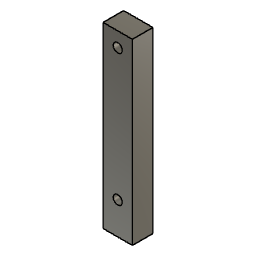
link2 v3 (Autodesk Fusion 360 design; units mm, degrees)
Autodesk Fusion 360 part; units mm, degrees
sketch "Sketch1" plane through (0, 0, 0) normal (0, 1, 0) x (1, 0, 0)
  line L0 (5, 27.5) -> (-5, 27.5)
  line L1 (-5, 27.5) -> (-5, -27.5)
  line L2 (-5, -27.5) -> (5, -27.5)
  line L3 (5, -27.5) -> (5, 27.5)
  line L4 (5, 27.5) -> (-5, -27.5) construction
  line L5 (-5, 27.5) -> (5, -27.5) construction
  line L6 (0, -24.05) -> (0, -22.5)
  circle A0 centre (0, -22.5) radius 1.55
  circle A1 centre (0, 22.5) radius 1.55
  dimension "d1" = 10
  dimension "d2" = 55
  dimension "d4" = 3.1
  constraint horizontal L0
  constraint perpendicular L0 L1
  constraint parallel L0 L2
  constraint parallel L1 L3
  constraint coincident L4 origin
  constraint coincident L5 origin
  constraint perpendicular L2 L6
  constraint coincident L6.end A0.centre
  constraint coincident A0 L6.start
  measures "d1" distance of L1.end L2.end
  measures "d2" distance of L0.end L1.end
  measures "d4" diameter of A0
extrude "Extrude1" add sketch "Sketch1" along normal blind 5
sketch "Sketch2" plane through (0, 0, -27.5) normal (0, 0, -1) x (1, 0, 0)
  line L0 (5, 0) -> (-5, 0)
  line L1 (-5, 0) -> (-5, -5)
  line L2 (-5, -5) -> (5, -5)
  line L3 (5, -5) -> (5, 0)
  circle A0 centre (0, -2.5) radius 1.75
  dimension "d7" = 2.5
  dimension "d8" = 3.5
  measures "d7" distance of origin A0.centre
  measures "d8" diameter of A0
extrude "Extrude2" cut sketch "Sketch2" against normal blind 2 contours A0
extrude "Extrude3" add 1 faces at (3.9167, 2.5, -27.5) along direction (0, 0, -1) blind 6
extrude "Extrude4" add 1 faces at (-0.3896, 1.8511, -25.5) along direction (0, 0, -1) blind 2
extrude "Extrude5" add 1 faces at (-0.0386, 5, -30.3486) along direction (0, 1, 0) blind 1
extrude "Extrude6" add 1 faces at (-0.0386, 0, -30.3486) along direction (0, -1, 0) blind 1
